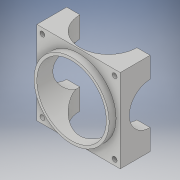
# Autodesk Inventor part: peca2
Saved by Autodesk Inventor 2019 (Build 230136000, 136)
## iProperties
Created: 2019-04-16
Part Number: peca2
Material: Generic
Document SubType Name: Modeling
Designer: Vladimir
Density: 1 g/cm^3
Appearance: Default
Author: Vladimir
Autodesk Inventor part; units mm, degrees
ref_plane "YZ Plane" through (0, 0, 0) normal (1, 0, 0) x (0, 1, 0)
ref_plane "XZ Plane" through (0, 0, 0) normal (0, 1, 0) x (-1, 0, 0)
ref_plane "XY Plane" through (0, 0, 0) normal (0, 0, 1) x (1, 0, 0)
sketch "Sketch1" plane through (0, 0, 0) normal (0, 0, 1) x (1, 0, 0)
  line L0 (-30, -30) -> (30, -30)
  line L1 (30, -30) -> (30, 30)
  line L2 (30, 30) -> (-30, 30)
  line L3 (-30, 30) -> (-30, -30)
  line L4 (-30, -30) -> (30, 30) construction
  line L5 (30, -30) -> (-30, 30) construction
  point P0 (0, 0)
  dimension "d0" = 60
  dimension "d1" = 60
  constraints: 12 end point, 2 midpoint, 2 parallel, 1 horizontal, 1 perpendicular
  measures "d0" distance of L0.end L1.end
  measures "d1" distance of L1.end L2.end
extrude "Extrusion1" add sketch "Sketch1" along normal blind 43
sketch "Sketch2" plane through (0, 0, 43) normal (0, 0, 1) x (1, 0, 0)
  circle A0 centre (0, 0) radius 25
  dimension "d4" = 50
  constraints: 1 centre point, 1 coincident
  measures "d4" diameter of A0
extrude "Extrusion2" cut sketch "Sketch2" against normal blind 43
sketch "Sketch3" plane through (30, -30, 0) normal (1, 0, 0) x (0, 0, -1)
  line L0 (0, 0) -> (0, 60) projected
  line L1 (0, 60) -> (-43, 60) projected
  line L2 (-43, 0) -> (-43, 60) projected
  line L3 (0, 0) -> (-43, 0) projected
  circle A0 centre (-21.5, 30) radius 15
  point P0 (0, 30)
  dimension "d7" = 30
  dimension "d8" = 21.5
  dimension "d9" = 30
  dimension "d10" = 60
  dimension "d11" = 43
  constraints: 1 centre point
  measures "d7" diameter of A0
  measures "d8" distance from line of A0.centre L0
  measures "d9" distance from line of L1 A0.centre
  measures "d10" distance of L0.start L0.end
  measures "d11" distance of L0.end L1.end
extrude "Extrusion3" cut sketch "Sketch3" against normal blind 430 contours A0
sketch "Sketch4" plane through (-30, 30, 0) normal (0, 1, 0) x (1, 0, 0)
  line L0 (60, 0) -> (0, 0) projected
  line L1 (0, 0) -> (0, -43) projected
  line L2 (60, -43) -> (0, -43) projected
  line L3 (60, 0) -> (60, -43) projected
  circle A0 centre (30, -21.5) radius 20.5
  point P0 (30, 0)
  dimension "d14" = 41
  dimension "d15" = 60
  dimension "d16" = 43
  dimension "d17" = 21.5
  dimension "d18" = 30
  constraints: 1 centre point
  measures "d14" diameter of A0
  measures "d15" distance of L0.start L0.end
  measures "d16" distance of L0.end L1.end
  measures "d17" distance from line of L0 A0.centre
  measures "d18" distance from line of A0.centre L1
extrude "Extrusion4" cut sketch "Sketch4" against normal blind 430 contours A0
sketch "Sketch5" plane through (0, 0, 43) normal (0, 0, 1) x (1, 0, 0)
  circle A0 centre (0, 0) radius 25 projected
  line L0 (-30, -30) -> (30, -30) projected
  line L1 (30, -30) -> (30, 30) projected
  line L2 (30, 30) -> (-30, 30) projected
  line L3 (-30, 30) -> (-30, -30) projected
  circle A1 centre (0, 0) radius 27
  dimension "d21" = 2
  constraints: 1 centre point, 1 coincident
  measures "d21" radial gap between concentric circles of A1 A0
extrude "Extrusion5" add sketch "Sketch5" along normal blind 5 contours A1
sketch "Sketch6" plane through (0, 0, 43) normal (0, 0, 1) x (1, 0, 0)
  circle A0 centre (0, 0) radius 27 projected
  line L0 (-30, -30) -> (30, -30) projected
  line L1 (30, -30) -> (30, 30) projected
  line L2 (30, 30) -> (-30, 30) projected
  line L3 (-30, 30) -> (-30, -30) projected
  circle A1 centre (-26, -26) radius 1.75
  dimension "d24" = 3.5
  dimension "d25" = 4
  dimension "d26" = 4
  constraints: 1 centre point
  measures "d24" diameter of A1
  measures "d25" distance from line of L0 A1.centre
  measures "d26" distance from line of A1.centre L3
extrude "Extrusion6" cut sketch "Sketch6" against normal blind 500 contours A1
pattern_circular "Circular Pattern1" count 4 over 360 about axis through (0, 0, 43) along (0, 0, -1) of "Extrusion6"
sketch "Sketch7" plane through (0, 0, 0) normal (0, 0, -1) x (-1, 0, 0)
  circle A0 centre (-26, -26) radius 1.75 projected
  circle A1 centre (-26, 26) radius 1.75 projected
  circle A2 centre (26, 26) radius 1.75 projected
  circle A3 centre (26, -26) radius 1.75 projected
  circle A4 centre (0, 0) radius 25 projected
  line L0 (30, -30) -> (-30, -30) projected
  line L1 (30, 30) -> (30, -30) projected
  line L2 (-30, 30) -> (30, 30) projected
  line L3 (-30, -30) -> (-30, 30) projected
  line L4 (49.4282, -48.51) -> (-49.4282, -48.51)
  line L5 (-49.4282, -48.51) -> (-49.4282, 48.51)
  line L6 (-49.4282, 48.51) -> (49.4282, 48.51)
  line L7 (49.4282, 48.51) -> (49.4282, -48.51)
  line L8 (49.4282, -48.51) -> (-49.4282, 48.51) construction
  line L9 (-49.4282, -48.51) -> (49.4282, 48.51) construction
  constraints: 12 end point, 2 midpoint, 2 parallel, 1 horizontal, 1 perpendicular
extrude "Extrusion7" cut sketch "Sketch7" against normal blind 21.5 contours A0 | A1 | A2 | A3 | A4 | L0 L3 L2 L1 | L4 L5 L6 L7
equation "\"d8\" = 0.5 * d11"
equation "\"d9\" = 0.5 * d10"
equation "\"d17\" = 0.5 * d16"
equation "\"d18\" = 0.5 * d15"
equation "\"d26\" = d25"
equation "\"d32\" = 0.5 * d2"
equation "\"d2\" = 43"
body "Solid1"
